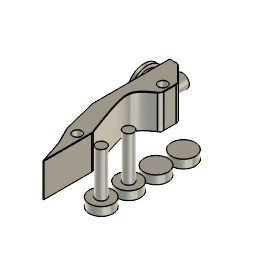
Balloon Car Original (Autodesk Fusion 360 design; units mm, degrees)
part number: 2025-09-21-17-09-51-574
Autodesk Fusion 360 part; units mm, degrees
sketch "Car Area" plane through (0, 0, 0) normal (0, 0, 1) x (1, 0, 0)
  line L0 (0, 30) -> (0, 45)
  line L1 (0, 0) -> (-15, 0)
  line L2 (-15, 0) -> (-15, 90)
  line L3 (-15, 90) -> (0, 90)
  line L4 (0, 90) -> (0, 0)
  circle A0 centre (-4, 25) radius 2.65
  circle A1 centre (-4, 75) radius 2.65
  line L5 (0, 0) -> (-5, 15)
  line L6 (-10, 25) -> (-15, 45)
  spline S0 degree 2 poles (0, 30) (-12, 62) (0, 70) knots 0 0 0 4.457712 4.457712 4.457712 weights 1 3 1
  line L7 (-5, 15) -> (-10, 25)
  line L8 (0, 80) -> (-10, 90)
  dimension "d4" = 15
  dimension "d5" = 90
  dimension "d6" = 15
  dimension "d7" = 90
  dimension "lol" = 5.3
  dimension "d11" = 5.3
  constraint coincident L1.start L4.end
  constraint perpendicular L1 L2
  constraint perpendicular L2 L3
  constraint perpendicular L1 L4
  constraint coincident L2 L6.end
  constraint coincident L4 S0.end
  constraint midpoint L2 L6.end
  constraint coincident L4 L8.start
  constraint coincident L3 L8.end
  constraint horizontal L3
  measures "d4" distance of L1.start L1.end
  measures "d5" distance of L1.end L2.end
  measures "d6" distance of L2.end L3.end
  measures "d7" distance of L3.end L1.start
  measures "lol" diameter of A0
  measures "d11" diameter of A1
extrude "Extrude1" add sketch "Car Area" along normal blind 20 contours L2 L3 L4 L5 L6 S0 L7 L8 makes body 1
sketch "Balloon Connector Start" plane through (-15, 0, 0) normal (-1, 0, 0) x (0, -1, 0)
  line L0 (-90, 0) -> (-45, 0)
  line L1 (-45, 0) -> (-45, 20)
  line L2 (-45, 20) -> (-90, 20)
  line L3 (-90, 20) -> (-90, 0)
  circle A0 centre (-80, 10) radius 8
extrude "Extrude2" add sketch "Balloon Connector Start" along normal blind 3 contours A0 bodies 1
sketch "Balloon Connector Mid" plane through (-18, 0, 0) normal (-1, 0, 0) x (0, -1, 0)
  circle A0 centre (-80, 10) radius 8
  circle A1 centre (-80, 10) radius 10
  dimension "d25" = 20
  constraint concentric A0 A1
  measures "d25" diameter of A1
extrude "Extrude3" add sketch "Balloon Connector Mid" along normal blind 2 contours A0 | A1 bodies 1
hole "Hole1" at (-20, 80, 10) direction (1, 0, 0) diameter 9 depth 9 tip angle 118 countersink diameter 16 countersink angle 90 bodies 1
sketch "Center for Balloon Connector Mouthpiece" plane through (0, 90, 0) normal (0, 1, 0) x (-1, 0, 0)
  line L0 (10, 0) -> (15, 0)
  line L1 (15, 0) -> (15, 20)
  line L2 (15, 20) -> (10, 20)
  line L3 (10, 20) -> (10, 0)
  line L4 (10, 0) -> (10, 10) construction
  constraint coincident L0.start L3.end
  constraint midpoint L3 L4.end
hole "Hole2" at (-10, 90, 10) direction (0, -1, 0) diameter 6 depth 9 tip angle 90 bodies 1
sketch "Balloon Connector Mouthpiece" plane through (0, 90, 0) normal (0, 1, 0) x (-1, 0, 0)
  arc A0 (10, 7) -> (10, 13) centre (10, 10) ccw
  line L0 (10, 7) -> (10, 0)
  line L1 (10, 0) -> (15, 0)
  line L2 (15, 0) -> (15, 20)
  line L3 (15, 20) -> (10, 20)
  line L4 (10, 20) -> (10, 13)
  circle A1 centre (10, 10) radius 4
  constraint concentric A0 A1
extrude "Extrude4" add sketch "Balloon Connector Mouthpiece" against normal blind 7 from surface at 3 thin wall 1 inside contours A0 L0 L4 A1 | A0 L0 L4 A1 bodies 1
fillet "Fillet1" radius 0.25 1 edges at (0, 0, 10) on bodies 1
fillet "Fillet2" radius 6 2 edges at (-10, 25, 10) (-15, 45, 10) on bodies 1
chamfer "Chamfer1" distance 0.25 distance2 0.25 23 edges at (-2.7436, 8.2308, 20) (-0.21, 1.2938, 20) (0, 15.7703, 20) (-7.3527, 19.7055, 20) (-15, 67.8693, 20) (-14.955, 45.0055, 20) (-12.4903, 34.9612, 20) (-9.9662, 25.0125, 20) (-9, 59, 20) (0, 75, 20) (-5, 85, 20) (-12.5, 90, 20) (-5, 85, 0) (-15, 67.8693, 0) (-7.3527, 19.7055, 0) (-9.9662, 25.0125, 0) (-12.4903, 34.9612, 0) (-14.955, 45.0055, 0) (0, 75, 0) (-9, 59, 0) (-2.7436, 8.2308, 0) (0, 15.7703, 0) (-0.21, 1.2938, 0) measured on face at (-7.7638, 43.0749, 20) measured on face at (-0.4347, 1.3721, 13.3333) measured on face at (-7.7638, 43.0749, 20) measured on face at (-7.7638, 43.0749, 20) measured on face at (-7.7638, 43.0749, 20) measured on face at (-14.8914, 44.6023, 6.6667) measured on face at (-7.7638, 43.0749, 20) measured on face at (-10.0822, 25.3579, 6.6667) measured on face at (-7.7638, 43.0749, 20) measured on face at (-7.7638, 43.0749, 20) measured on face at (-7.7638, 43.0749, 20) measured on face at (-7.7638, 43.0749, 20) measured on face at (-2.0011, 82.0011, 9.9467) measured on face at (-7.7638, 43.0749, 0) measured on face at (-7.7638, 43.0749, 0) measured on face at (-10.0822, 25.3579, 6.6667) measured on face at (-7.7638, 43.0749, 0) measured on face at (-14.8914, 44.6023, 6.6667) measured on face at (-7.7638, 43.0749, 0) measured on face at (-1.7549, 34.7075, 8.3333) measured on face at (-7.7638, 43.0749, 0) measured on face at (-7.7638, 43.0749, 0) measured on face at (-0.4347, 1.3721, 13.3333) on bodies 1
fillet "Fillet3" radius 2 1 edges at (-15, 87.4586, 12.8929) on bodies 1
fillet "Fillet4" radius 3 5 edges at (0, 30, 10) (0, 70, 10) (0, 80, 10) (-10, 90, 16.875) (-10, 90, 3.125) on bodies 1
fillet "Fillet5" radius 0.5 2 edges at (-6.2707, 93, 8.5535) (-7.203, 93, 11.0848) on bodies 1
sketch "Wheels" plane through (0, 0, 0) normal (0, 0, 1) x (1, 0, 0)
  circle A0 centre (20, 15) radius 3
  circle A1 centre (20, 40) radius 7
  circle A2 centre (20, 15) radius 7
  dimension "d52" = 14
  dimension "d53" = 14
  constraint concentric A0 A2
  measures "d52" diameter of A1
  measures "d53" diameter of A2
extrude "Extrude5" add sketch "Wheels" along normal blind 5 separate body contours A0 | A2 makes body 2
extrude "Extrude6" add sketch "Wheels" along normal blind 31 contours A0 bodies 2
extrude "Extrude7" add sketch "Wheels" along normal blind 5 separate body contours A1 makes body 3
move_body "Move1" bodies 3 to x (1, 0, 0) y (0, 1, 0) z (0, 0, 1) at (0, 17, 0)
copy_body "CopyPasteBodies1" bodies 2 makes body 4
move_body "Move2" bodies 4 to x (1, 0, 0) y (0, 1, 0) z (0, 0, 1) at (0, 16, 0)
move_body "Move3" bodies 3 to x (1, 0, 0) y (0, 1, 0) z (0, 0, 1) at (0, -10, 0)
copy_body "CopyPasteBodies2" bodies 3 makes body 5
move_body "Move4" bodies 5 to x (1, 0, 0) y (0, 1, 0) z (0, 0, 1) at (0, 16, 0)
equation "d4 = CarHeight"
equation "d5 = CarLength"
equation "d6 = CarHeight"
equation "d7 = CarLength"
equation "lol = AxleWidth + AxleOffset"
equation "d11 = AxleWidth + AxleOffset"
equation "AxleWidth = 5 mm"
equation "AxleOffset = 0.3 mm"
equation "CarLength = 90 mm"
equation "CarHeight = 15 mm"
equation "CarWidth = 20 mm"
equation "WheelThickness = 5 mm"
equation "WheelDiameter = 14 mm"
equation "AxleLength = CarWidth + 1 mm + ( WheelThickness * 2 )"
equation "d21 = CarWidth"
equation "d52 = WheelDiameter"
equation "d53 = WheelDiameter"
equation "d54 = WheelThickness"
equation "d56 = AxleLength"
equation "d58 = WheelThickness"
named bodies: "Chassis", "Axle 1", "Wheel 1", "Axle 2", "Wheel 2"
